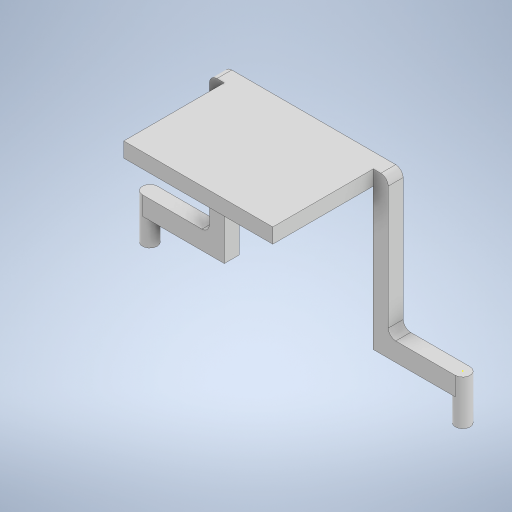
# Autodesk Inventor part: recubrimiento de motor
Saved by Autodesk Inventor 2024.3 (Build 283343000, 343)
## iProperties
Created: 2024-05-16
Part Number: recubrimiento de motor
Material: Generic
Document SubType Name: Modeling
Designer: JDAM
Density: 1 g/cm^3
Appearance: Default
Author: JDAM
Autodesk Inventor part; units mm, degrees
ref_plane "YZ Plane" through (0, 0, 0) normal (1, 0, 0) x (0, 1, 0)
ref_plane "XZ Plane" through (0, 0, 0) normal (0, 1, 0) x (-1, 0, 0)
ref_plane "XY Plane" through (0, 0, 0) normal (0, 0, 1) x (1, 0, 0)
sketch "Sketch1" plane through (0, 0, 0) normal (0, 1, 0) x (-1, 0, 0)
  circle A0 centre (0, 0) radius 2
  line L0 (0, 2) -> (22, 2)
  line L1 (22, 2) -> (22, -2)
  line L2 (22, 2) -> (22, 29)
  line L3 (22, 29) -> (62, 29)
  line L4 (22, -2) -> (62, -2)
  line L5 (62, 29) -> (62, -2)
  line L6 (17.9896, 2) -> (17.9896, -2)
  line L7 (62, -2) -> (62, 2)
  line L8 (22, -2) -> (0, -2)
  line L9 (62, 2) -> (84, 2)
  line L10 (62, -2) -> (84, -2)
  circle A1 centre (84, 0) radius 2
  line L11 (66.01, 2) -> (66.01, -2)
  line L12 (66.01, 2) -> (62, 2)
  line L13 (62, -2) -> (66.01, -2)
  line L14 (17.9896, 2) -> (22, 2)
  line L15 (22, -2) -> (17.9896, -2)
  line L16 (66.01, 2) -> (66.01, -2)
  line L17 (62, -2) -> (62, 2)
  line L18 (17.9896, -2) -> (17.9896, 2)
  line L19 (22, 2) -> (22, -2)
  line L20 (66.01, 2) -> (66.01, -2)
  line L21 (62, -2) -> (62, 2)
  line L22 (22, -2) -> (22, 2)
  line L23 (22, -2) -> (22, 2)
  line L24 (22, 2) -> (22, -2)
  line L25 (17.9896, -2) -> (17.9896, 2)
  line L26 (62, 2) -> (66.01, 2)
  line L27 (66.01, -2) -> (62, -2)
  line L28 (22, 2) -> (22, -2)
  line L29 (17.9896, -2) -> (17.9896, 2)
  line L30 (22, 2) -> (17.9896, 2)
  line L31 (22, -2) -> (17.9896, -2)
  line L32 (66.01, 2) -> (62, 2)
  line L33 (62, -2) -> (62, 2)
  line L34 (66.01, -2) -> (62, -2)
  line L35 (66.01, 2) -> (66.01, -2)
  dimension "d0" = 4
  dimension "d8" = 4
  dimension "d9" = 22
  dimension "d13" = 4
  dimension "d16" = 4.01
  constraints: 72 end point, 9 parallel, 9 vertical, 8 horizontal, 5 perpendicular, 5 point on line, 2 centre point, 2 collinear, 2 point on circle, 1 coincident
  measures "d0" diameter of A0
  measures "d8" distance of L4.end L7.end
  measures "d9" distance of L7.end L9.end
  measures "d13" diameter of A1
  measures "d16" distance of L7.end L11.start
extrude "Extrusion1" add sketch "Sketch1" against normal blind 7 contours A0 | A1
extrude "Extrusion2" add sketch "Sketch1" along normal blind 5 contours A0 | A0 L0 L6 L8 | L11 L9 A1 L10 | A1
sketch "Sketch2" plane through (0, 5, 0) normal (0, 1, 0) x (1, 0, 0)
  point P0 (0, 0)
extrude "Extrusion3" add sketch "Sketch1" along normal blind 42 contours L0 L1 L8 L6 | L5 L9 L11 L10
extrude "Extrusion4" add sketch "Sketch1" along normal blind 42 contours L2 L3 L5 L4 L1
extrude "Extrusion5" cut sketch "Sketch1" along normal blind 38 contours L2 L3 L5 L4 L1
fillet "Fillet1" radius 2 4 edges at (-66.01, 5, 0) (-66.01, 42, 0) (-17.9896, 42, 0) (-17.9896, 5, 0)
body "Solid1"
